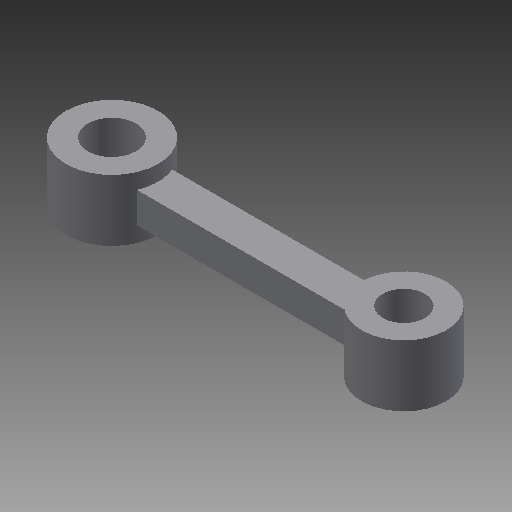
# Autodesk Inventor part: Crank Arm
Saved by Autodesk Inventor 2017 (Build 210142000, 142)
## iProperties
Created: 2012-08-14
Part Number: Crank Arm
Material: Generic
Document SubType Name: Modeling
Designer: John
Density: 1 g/cm^3
Appearance: Default
Author: John
Autodesk Inventor part; units mm, degrees
ref_plane "YZ Plane" through (0, 0, 0) normal (1, 0, 0) x (0, 1, 0)
ref_plane "XZ Plane" through (0, 0, 0) normal (0, 1, 0) x (-1, 0, 0)
ref_plane "XY Plane" through (0, 0, 0) normal (0, 0, 1) x (1, 0, 0)
sketch "Sketch1" plane through (0, 0, 0) normal (0, 0, 1) x (1, 0, 0)
  circle A0 centre (0, 0) radius 3.81
  circle A1 centre (24.13, 0) radius 3.4925
  line L0 (0, 1.4605) -> (24.13, 1.4605)
  line L1 (24.13, 1.4605) -> (24.13, -1.4605)
  line L2 (24.13, -1.4605) -> (0, -1.4605)
  line L3 (0, -1.4605) -> (0, 1.4605)
  dimension "d0" = 7.62
  dimension "d1" = 2.921
  dimension "d2" = 1.4605
  dimension "d3" = 24.13
  dimension "d15" = 6.985
  constraints: 8 end point, 2 centre point, 2 coincident, 2 parallel, 2 vertical alignment, 1 horizontal, 1 horizontal alignment, 1 midpoint, 1 perpendicular
  measures "d0" diameter of A0
  measures "d1" distance of L0.end L1.end
  measures "d2" distance from line of A1.centre L0
  measures "d3" distance of A1.centre A0.centre
  measures "d15" diameter of A1
extrude "Extrusion1" add sketch "Sketch1" along normal mid plane 5.08 contours A0 L2 L3 L0 | L0 L3 L2 A0 | L0 L1 L2 A1 | A1 L2 L1 L0
extrude "Extrusion2" add sketch "Sketch1" along normal mid plane 2.54 contours A0 L2 L3 L0 | A0 L0 A1 L2 | L0 L1 L2 A1 picked at (1.27, 0) picked at (22.9658, 0)
hole "Hole2" at (0, 0, 2.54) direction (0, 0, -1) diameter 3.9878 end through all
hole "Hole3" at (24.13, 0, 2.54) direction (0, 0, -1) diameter 3.4798 end through all
equation "\"d2\" = 0.5 * d1"
body "Solid1"
